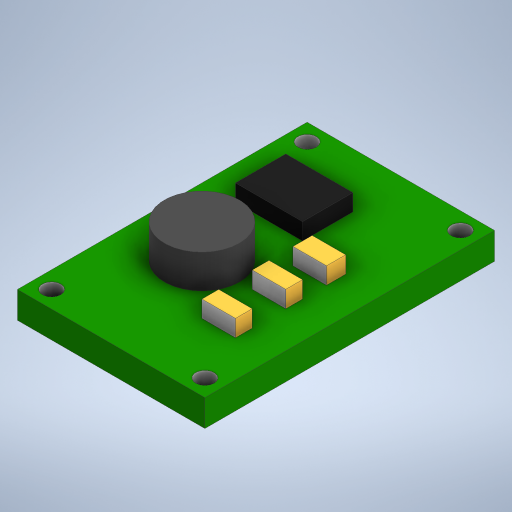
# Autodesk Inventor part: MH-MINI-360
Saved by Autodesk Inventor 2023 (Build 270158000, 158)
## iProperties
Created: 2024-02-24
Part Number: MH-MINI-360
Material: Ogólny
Document SubType Name: Modeling
Designer: Kamil
Density: 1 g/cm^3
Appearance: Domyślna
Author: Kamil
Autodesk Inventor part; units mm, degrees
ref_plane "YZ Plane" through (0, 0, 0) normal (1, 0, 0) x (0, 1, 0)
ref_plane "XZ Plane" through (0, 0, 0) normal (0, 1, 0) x (-1, 0, 0)
ref_plane "XY Plane" through (0, 0, 0) normal (0, 0, 1) x (1, 0, 0)
sketch "Szkic1" plane through (0, 0, 0) normal (0, 1, 0) x (-1, 0, 0)
  line L0 (0, 0) -> (-11.176, 0)
  line L1 (-11.176, 0) -> (-11.176, -17.272)
  line L2 (-11.176, -17.272) -> (0, -17.272)
  line L3 (0, -17.272) -> (0, 0)
  dimension "d0" = 17.272
  dimension "d1" = 11.176
  constraints: 8 end point, 2 parallel, 1 horizontal, 1 perpendicular
  measures "d0" distance of L2.end L0.start
  measures "d1" distance of L0.start L0.end
extrude "Wyciągnięcie proste1" add sketch "Szkic1" along normal blind 1.6
sketch "Szkic2" plane through (0, 1.6, 0) normal (0, 1, 0) x (1, 0, 0)
  line L0 (11.176, 0) -> (11.176, 17.272) projected
  line L1 (11.176, 17.272) -> (0, 17.272) projected
  line L2 (0, 17.272) -> (0, 0) projected
  line L3 (0, 0) -> (11.176, 0) projected
  circle A0 centre (1.016, 1.016) radius 0.55
  circle A1 centre (1.016, 16.256) radius 0.55
  circle A2 centre (10.16, 1.016) radius 0.55
  circle A3 centre (10.16, 16.256) radius 0.55
  line L4 (1.016, 1.016) -> (1.016, 16.256)
  line L5 (1.016, 16.256) -> (10.16, 16.256)
  point P0 (1.016, 8.636)
  point P1 (0, 8.636)
  point P2 (5.588, 16.256)
  point P3 (5.588, 17.272)
  dimension "d4" = 1.1
  dimension "d5" = 1.1
  dimension "d6" = 1.1
  dimension "d7" = 1.1
  dimension "d8" = 15.24
  dimension "d9" = 9.144
  constraints: 4 centre point, 4 end point, 4 midpoint, 3 horizontal alignment, 3 vertical alignment, 1 horizontal, 1 vertical
  measures "d4" diameter of A0
  measures "d5" diameter of A1
  measures "d6" diameter of A2
  measures "d7" diameter of A3
  measures "d8" distance of L4.start L4.end
  measures "d9" distance between centres of A3 A1
extrude "Wyciągnięcie proste2" cut sketch "Szkic2" against normal through all contours A0 | A3 | A1 L5 L4 | L4 L5 A1 | A2
sketch "Szkic3" plane through (0, 1.6, 0) normal (0, 1, 0) x (1, 0, 0)
  circle A0 centre (4, 7) radius 2.2361
  line L0 (7, 4) -> (9, 4)
  line L1 (9, 4) -> (9, 5)
  line L2 (9, 5) -> (7, 5)
  line L3 (7, 5) -> (7, 4)
  line L4 (7, 7) -> (9, 7)
  line L5 (9, 7) -> (9, 8)
  line L6 (9, 8) -> (7, 8)
  line L7 (7, 8) -> (7, 7)
  line L8 (7, 9.4289) -> (9, 9.4289)
  line L9 (9, 9.4289) -> (9, 10.5737)
  line L10 (9, 10.5737) -> (7, 10.5737)
  line L11 (7, 10.5737) -> (7, 9.4289)
  line L12 (2, 11) -> (6, 11)
  line L13 (6, 11) -> (6, 14)
  line L14 (6, 14) -> (2, 14)
  line L15 (2, 14) -> (2, 11)
  point P0 (0, 0)
  constraints: 32 end point, 8 parallel, 4 horizontal, 4 perpendicular, 2 point on line, 1 centre point
extrude "Wyciągnięcie proste3" add sketch "Szkic3" along normal blind 1
extrude "Wyciągnięcie proste4" add sketch "Szkic3" along normal blind 2 contours A0
